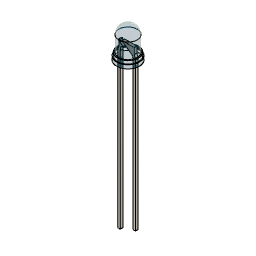
3mm T1 v6 (Autodesk Fusion 360 design; units mm, degrees)
Autodesk Fusion 360 part; units mm, degrees
sketch "Sketch2" plane through (0, 0, 0) normal (0, 0, 1) x (1, 0, 0)
  circle A0 centre (0, 0) radius 1.75
  circle A1 centre (0, 0) radius 1.9
  circle A2 centre (0, 0) radius 1.55
  dimension "d8" = 3.5
  dimension "d9" = 3.8
  dimension "d10" = 3.1
  constraint coincident A0.centre A1.centre
  constraint concentric A0 A2
  measures "d8" diameter of A0
  measures "d9" diameter of A1
  measures "d10" diameter of A2
extrude "Extrude1" add sketch "Sketch2" along normal blind 5.2 contours A2 makes body 1
fillet "Fillet1" radius 1.55 1 edges at (-1.4451, -0.5605, 5.2) on bodies 1
extrude "Extrude2" add sketch "Sketch2" along normal blind 1.1 contours A0 bodies 1
extrude "Extrude3" add sketch "Sketch2" along normal blind 0.6 contours A1 bodies 1
copy_body "CutPasteBodies1" bodies 1 removing the originals makes body 2 in component "Lense"
sketch "Sketch3" plane through (0, 0, 0) normal (0, 0, 1) x (1, 0, 0)
  line L0 (-1.07, 0.225) -> (-1.47, 0.225)
  line L1 (-1.47, 0.225) -> (-1.47, -0.225)
  line L2 (-1.47, -0.225) -> (-1.07, -0.225)
  line L3 (-1.07, -0.225) -> (-1.07, 0.225)
  line L4 (-1.07, 0.225) -> (-1.47, -0.225) construction
  line L5 (-1.47, 0.225) -> (-1.07, -0.225) construction
  line L6 (1.47, 0.225) -> (1.07, 0.225)
  line L7 (1.07, 0.225) -> (1.07, -0.225)
  line L8 (1.07, -0.225) -> (1.47, -0.225)
  line L9 (1.47, -0.225) -> (1.47, 0.225)
  line L10 (1.47, 0.225) -> (1.07, -0.225) construction
  line L11 (1.07, 0.225) -> (1.47, -0.225) construction
  point P0 (-1.27, 0)
  point P1 (1.27, 0)
  dimension "d19" = 1.27
  dimension "d20" = 1.27
  dimension "d27" = 0.4
  dimension "d28" = 0.45
  dimension "d29" = 0.4
  dimension "d30" = 0.45
  constraint horizontal L0
  constraint perpendicular L0 L1
  constraint parallel L0 L2
  constraint parallel L1 L3
  constraint coincident L4 P0
  constraint coincident L5 P0
  constraint horizontal L6
  constraint perpendicular L6 L7
  constraint parallel L6 L8
  constraint parallel L7 L9
  constraint coincident L10 P1
  constraint coincident L11 P1
  measures "d19" distance of origin P1
  measures "d20" distance of origin P0
  measures "d27" distance of L1.end L2.end
  measures "d28" distance of L0.end L1.end
  measures "d29" distance of L7.end L8.end
  measures "d30" distance of L6.end L7.end
extrude "Extrude4" add sketch "Sketch3" against normal blind 24 separate body makes body 3 at (-1.07, -0.075, -8) makes body 4 at (1.47, -0.075, -8)
copy_body "CutPasteBodies1'" bodies 3 removing the originals makes body 5 in component "Pins"
copy_body "CutPasteBodies2" bodies 4 removing the originals makes body 6 in component "Pins"
extrude "Extrude1'" add 1 faces at (-1.2033, -0.075, -24) along direction (0, 0, -1) blind 1 on bodies 5 bodies 5 in component "Pins"
extrude "Extrude2'" add 2 faces at (-1.2033, -0.075, 0) (1.2033, 0.075, 0) along direction (0, 0, 1) blind 0.9 on bodies 5 6 bodies 5 6 in component "Pins"
sketch "Sketch4" plane through (0, -0.225, 0) normal (0, -1, 0) x (1, 0, 0)
  line L0 (1.07, 0.9) -> (1.07, -24)
  line L1 (1.07, -24) -> (1.47, -24)
  line L2 (1.47, -24) -> (1.47, 0.9)
  line L3 (1.47, 0.9) -> (1.07, 0.9)
  line L4 (1.47, 0.9) -> (1.27, 1.4813)
  line L5 (1.27, 1.4813) -> (1.27, 2.5)
  line L6 (1.27, 2.5) -> (-0.8, 2.5)
  line L7 (-0.8, 2.5) -> (0.9909, 1.1907)
  line L8 (0.9909, 1.1907) -> (1.07, 0.9)
  line L9 (1.47, 0.9) -> (1.07, 0.9)
  line L10 (-1.47, 0.9) -> (-1.3, 1.5)
  line L11 (-1.3, 1.5) -> (-1.3, 2.5)
  line L12 (-1.3, 2.5) -> (-1.1, 2.5)
  line L13 (-1.1, 2.5) -> (-1.1, 2.1)
  line L14 (-1.1, 2.1) -> (-0.6, 1.7)
  line L15 (-0.6, 1.7) -> (-1, 1.5)
  line L16 (-1, 1.5) -> (-1.07, 0.9)
  line L17 (-1.07, 0.9) -> (-1.47, 0.9)
  constraint coincident L2.end L3.start
  constraint perpendicular L3 L5
  constraint perpendicular L0 L6
  constraint coincident L0.start L3.end
  constraint vertical L11
  constraint perpendicular L11 L12
  constraint perpendicular L12 L13
  constraint horizontal L17
extrude "Extrude3'" add sketch "Sketch4" against normal blind 0.45 contours L3 L4 L5 L6 L7 L8 L9 bodies 6 in component "Pins"
extrude "Extrude4'" add sketch "Sketch4" against normal blind 0.45 contours L10 L11 L12 L13 L14 L15 L16 L17 bodies 5 in component "Pins"
component "Lense" placed x (1, 0, 0) y (0, 1, 0) z (0, 0, 1) at (0, 0, 0)
component "Pins" placed x (1, 0, 0) y (0, 1, 0) z (0, 0, 1) at (0, 0, 0)
